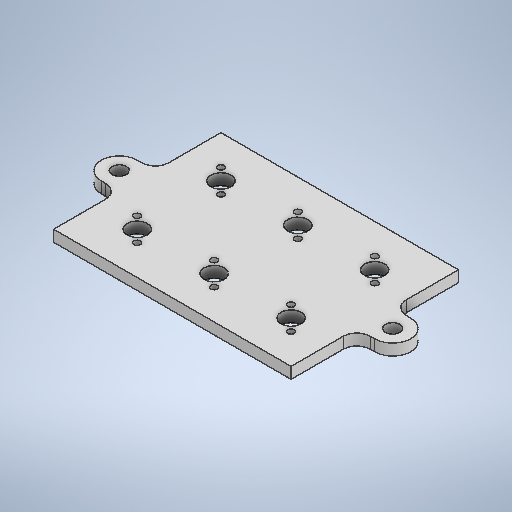
# Autodesk Inventor part: Part6
Saved by Autodesk Inventor 2025.1 (Build 291241000, 241)
## iProperties
Created: 2025-02-27
Part Number: Part6
Material: Generic
Document SubType Name: Modeling
Designer: santiago
Density: 1 g/cm^3
Appearance: Default
Author: santiago
Autodesk Inventor part; units mm, degrees
ref_plane "YZ Plane" through (0, 0, 0) normal (1, 0, 0) x (0, 1, 0)
ref_plane "XZ Plane" through (0, 0, 0) normal (0, 1, 0) x (-1, 0, 0)
ref_plane "XY Plane" through (0, 0, 0) normal (0, 0, 1) x (1, 0, 0)
sketch "Sketch1" plane through (0, 0, 0) normal (0, 1, 0) x (-1, 0, 0)
  arc A0 (27.5033, -3.6329) -> (24.5033, -6.6329) centre (27.5033, -6.6329) ccw
  arc A1 (28.5033, -3.6329) -> (28.5033, 4.3671) centre (28.5033, 0.3671) ccw
  line L0 (27.5033, -3.6329) -> (28.5033, -3.6329)
  line L1 (28.5033, 4.3671) -> (27.5033, 4.3671)
  arc A2 (24.5033, 7.3671) -> (27.5033, 4.3671) centre (27.5033, 7.3671) ccw
  line L2 (24.5033, 18.9671) -> (24.5033, 7.3671)
  line L3 (-28.2967, 18.9671) -> (24.5033, 18.9671)
  line L4 (-28.2967, 7.3671) -> (-28.2967, 18.9671)
  arc A3 (-31.2967, 4.3671) -> (-28.2967, 7.3671) centre (-31.2967, 7.3671) ccw
  line L5 (-31.2967, 4.3671) -> (-32.2967, 4.3671)
  arc A4 (-32.2967, 4.3671) -> (-32.2967, -3.6329) centre (-32.2967, 0.3671) ccw
  line L6 (-32.2967, -3.6329) -> (-31.2967, -3.6329)
  arc A5 (-28.2967, -6.6329) -> (-31.2967, -3.6329) centre (-31.2967, -6.6329) ccw
  line L7 (-28.2967, -18.2329) -> (-28.2967, -6.6329)
  line L8 (24.5033, -18.2329) -> (-28.2967, -18.2329)
  line L9 (24.5033, -6.6329) -> (24.5033, -18.2329)
  circle A6 centre (28.5033, 0.3671) radius 1.6
  circle A7 centre (-32.2967, 0.3671) radius 1.6
  circle A8 centre (-1.8967, 9.6671) radius 2.25
  circle A9 centre (15.2033, 9.6671) radius 2.25
  circle A10 centre (15.2033, -8.9329) radius 2.25
  circle A11 centre (-1.8967, -8.9329) radius 2.25
  circle A12 centre (-18.9967, -8.9329) radius 2.25
  circle A13 centre (-18.9967, 9.6671) radius 2.25
  point P0 (0, 0)
  constraints: 20 end point, 14 centre point, 12 point on circle
extrude "Extrusion1" add sketch "Sketch1" along normal blind 2.5
sketch "Sketch2" plane through (0, 2.5, 0) normal (0, 1, 0) x (1, 0, 0)
  line L0 (-12.6033, -12.2671) -> (-17.8033, -12.2671) construction
  line L1 (-17.8033, -12.2671) -> (-17.8033, -7.0671) construction
  line L2 (-17.8033, -7.0671) -> (-12.6033, -7.0671) construction
  line L3 (-12.6033, -7.0671) -> (-12.6033, -12.2671) construction
  circle A0 centre (-15.2033, -9.6671) radius 2.25 construction
  line L4 (-12.6033, -12.2671) -> (-17.8033, -7.0671) construction
  line L5 (-17.8033, -12.2671) -> (-12.6033, -7.0671) construction
  circle A1 centre (-17.8033, -7.0671) radius 0.75
  circle A2 centre (-12.6033, -12.2671) radius 0.75
  circle A3 centre (-17.8033, 11.5329) radius 0.75
  circle A4 centre (-12.6033, 6.3329) radius 0.75
  circle A5 centre (-0.7033, -7.0671) radius 0.75
  circle A6 centre (4.4967, -12.2671) radius 0.75
  circle A7 centre (-0.7033, 11.5329) radius 0.75
  circle A8 centre (4.4967, 6.3329) radius 0.75
  circle A9 centre (16.3967, -7.0671) radius 0.75
  circle A10 centre (21.5967, -12.2671) radius 0.75
  circle A11 centre (16.3967, 11.5329) radius 0.75
  circle A12 centre (21.5967, 6.3329) radius 0.75
  point P0 (0, 0)
  dimension "d2" = 1.5
  dimension "d3" = 1.5
  dimension "d6" = 18.6
  dimension "d9" = 17.1
  dimension "d14" = 5.2
  dimension "d15" = 5.2
  constraints: 12 centre point, 12 end point, 2 coincident, 2 horizontal, 2 midpoint, 2 parallel, 1 perpendicular, 1 vertical, 20 other
  measures "d2" diameter of A1
  measures "d3" diameter of A2
  measures "d6" distance of A1.centre A3.centre
  measures "d9" distance of A1.centre A5.centre
  measures "d14" distance of L2.end L0.start
  measures "d15" distance of L1.end L2.end
extrude "Extrusion2" cut sketch "Sketch2" against normal through all
equation "\"d3\" = d2"
body "Solid1"
